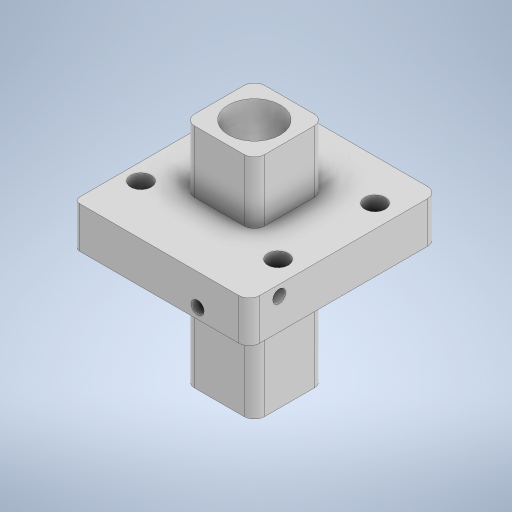
# Autodesk Inventor part: Contracting Finger Motion Motot Mount
Saved by Autodesk Inventor 2023.1 (Build 271208000, 208)
## iProperties
Created: 2022-12-19
Part Number: Contracting Finger Motion Motot Mount
Material: Generic
Document SubType Name: Modeling
Designer: shubh
Density: 1 g/cm^3
Appearance: Default
Author: shubh
Autodesk Inventor part; units mm, degrees
ref_plane "YZ Plane" through (0, 0, 0) normal (1, 0, 0) x (0, 1, 0)
ref_plane "XZ Plane" through (0, 0, 0) normal (0, 1, 0) x (-1, 0, 0)
sketch "Sketch1" plane through (0, 0, 0) normal (0, 1, 0) x (-1, 0, 0)
  line L0 (-57.15, 32.9184) -> (-57.15, -64.5668)
  line L1 (50.8, -30.5816) -> (50.8, 32.9184)
  line L2 (50.8, -43.8912) -> (50.8, -30.5816)
  circle A0 centre (40.3352, -58.0517) radius 6.35
  line L3 (-57.15, -45.1739) -> (-57.15, -83.2739)
  line L4 (-57.15, -83.2739) -> (50.8, -83.2739)
  line L5 (50.8, -83.2739) -> (50.8, -43.8912)
  line L6 (-57.15, 32.9184) -> (50.8, 32.9184)
  circle A1 centre (40.3352, 2.1209) radius 6.35
  circle A2 centre (-43.4848, -58.1279) radius 6.35
  circle A3 centre (-43.4848, 1.5367) radius 6.35
  point P0 (-6.35, 83.3882)
  dimension "d93" = 12.7
  dimension "d94" = 10.4648
  dimension "d96" = 25.2222
  dimension "d109" = 63.5
  dimension "d110" = 39.3827
  dimension "d111" = 13.3096
  dimension "d112" = 12.7
  dimension "d113" = 60.1726
  dimension "d115" = 12.7
  dimension "d116" = 83.82
  dimension "d117" = 25.146
  dimension "d118" = 12.7
  dimension "d119" = 59.6646
  dimension "d120" = 107.95
  dimension "d121" = 107.95
  constraints: 14 end point, 4 centre point, 2 parallel, 1 perpendicular
  measures "d93" diameter of A0
  measures "d94" distance from line of L1 A0.centre
  measures "d96" distance from line of A0.centre L4
  measures "d109" distance of L1.start L1.end
  measures "d110" distance of L4.end L2.start
  measures "d111" distance of L2.start L1.start
  measures "d112" diameter of A1
  measures "d113" distance of A1.centre A0.centre
  measures "d115" diameter of A2
  measures "d116" distance of A0.centre A2.centre
  measures "d117" distance from line of L4 A2.centre
  measures "d118" diameter of A3
  measures "d119" distance of A3.centre A2.centre
  measures "d120" distance of L3.end L4.end
  measures "d121" distance of L0.start L1.end
extrude "Extrusion1" add sketch "Sketch1" along normal blind 25.4
sketch "Sketch2" plane through (0, 25.4, 0) normal (0, 1, 0) x (1, 0, 0)
  line L0 (-21.59, 48.9458) -> (21.59, 48.9458)
  line L1 (21.59, 48.9458) -> (21.59, 5.7658)
  line L2 (21.59, 5.7658) -> (-21.59, 5.7658)
  line L3 (-21.59, 5.7658) -> (-21.59, 48.9458)
  line L4 (63.5, 61.6458) -> (-50.8, 61.6458) projected
  point P0 (0, 0)
  point P1 (-21.59, 27.3558)
  dimension "d15" = 43.18
  dimension "d80" = 12.7
  constraints: 8 end point, 2 parallel, 1 horizontal, 1 midpoint, 1 perpendicular
  measures "d15" distance of L0.end L1.end
  measures "d80" distance between parallel lines of L4 L0
extrude "Extrusion2" add sketch "Sketch2" along normal blind 38.1 and the other way blind 101.6
sketch "Sketch3" plane through (0, 63.5, 0) normal (0, 1, 0) x (1, 0, 0)
  circle A0 centre (0, 27.3558) radius 16.002
  line L0 (21.59, 48.9458) -> (-21.59, 48.9458) projected
  point P0 (0, 0)
  dimension "d81" = 32.004
  dimension "d82" = 21.59
  constraints: 1 centre point
  measures "d81" diameter of A0
  measures "d82" distance from line of L0 A0.centre
extrude "Extrusion3" cut sketch "Sketch3" against normal blind 50.8
ref_plane "Work Plane1" through (0, 17.78, 0) normal (0, 1, 0) x (1, 0, 0)
sketch "Sketch4" plane through (0, 17.78, 0) normal (0, 1, 0) x (1, 0, 0)
  circle A0 centre (0, 26.9875) radius 18.7452
  point P0 (0, 0)
  dimension "d85" = 37.4904
  constraints: 1 centre point
  measures "d85" diameter of A0
extrude "Extrusion4" cut sketch "Sketch4" against normal blind 76.2
fillet "Fillet1" radius 6.35 4 edges at (21.59, 44.45, -5.7658) (21.59, 44.45, -48.9458) (-21.59, 44.45, -5.7658) (-21.59, 44.45, -48.9458)
fillet "Fillet3" radius 3.175 1 edges at (-50.8, 12.7, 32.9184)
sketch "Sketch5" plane through (-50.8, 0, -58.4708) normal (-1, 0, 0) x (0, 0, 1)
  circle A0 centre (73.025, 19.05) radius 3.9751
  line L0 (-24.8031, 25.4) -> (88.2142, 25.4) projected
  line L1 (-3.175, 25.4) -> (-3.175, 0) projected
  point P0 (58.4708, 0)
  point P1 (0, 25.4)
  point P2 (-3.175, 12.7)
  point P3 (3.0734, 25.4)
  dimension "d66" = 7.9502
  dimension "d67" = 6.35
  dimension "d114" = 76.2
  constraints: 1 centre point, 1 midpoint
  measures "d66" diameter of A0
  measures "d67" distance from line of L0 A0.centre
  measures "d114" distance from line of L1 A0.centre
extrude "Extrusion5" cut sketch "Sketch5" against normal blind 254
sketch "Sketch6" plane through (-53.975, 0, 32.9184) normal (0, 0, 1) x (1, 0, 0)
  circle A0 centre (79.375, 6.35) radius 3.9751
  line L0 (111.125, 0) -> (111.125, 25.4) projected
  line L1 (0, 25.4) -> (107.95, 25.4) projected
  point P0 (53.975, 0)
  point P1 (111.125, 12.7)
  point P2 (53.975, 25.4)
  dimension "d71" = 7.9502
  dimension "d73" = 19.05
  dimension "d79" = 31.75
  constraints: 2 midpoint, 1 centre point
  measures "d71" diameter of A0
  measures "d73" vertical distance of point (53.975, 25.4) A0.centre
  measures "d79" horizontal distance of point (111.125, 12.7) A0.centre
extrude "Extrusion6" cut sketch "Sketch6" against normal blind 152.4
fillet "Fillet4" radius 6.35 4 edges at (-21.59, -38.1, -5.7658) (-21.59, -38.1, -48.9458) (21.59, -38.1, -5.7658) (21.59, -38.1, -48.9458)
fillet "Fillet5" radius 6.35 2 edges at (57.15, 12.7, 32.9184) (57.15, 12.7, -83.2739)
body "Solid1"
